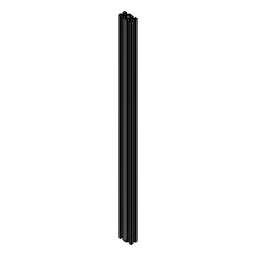
drawing-machine (Autodesk Fusion 360 archive; units mm, degrees)
design "40x20 extrusion"
Autodesk Fusion 360 part; units mm, degrees
sketch "Sketch1" plane through (0, 0, 0) normal (0, 0, 1) x (1, 0, 0)
  line L0 (20, -10) -> (-20, -10) construction
  line L1 (-20, -10) -> (-20, 10) construction
  line L2 (-20, 10) -> (20, 10) construction
  line L3 (20, 10) -> (20, -10) construction
  line L4 (20, -10) -> (-20, 10) construction
  line L5 (-20, -10) -> (20, 10) construction
  line L6 (0, -10) -> (0, 10) construction
  line L7 (-20, 0) -> (0, 0) construction
  circle A0 centre (-10, 0) radius 2.5
  line L8 (-6.1, -3.9) -> (-13.9, -3.9)
  line L9 (-13.9, -3.9) -> (-13.9, 3.9)
  line L10 (-13.9, 3.9) -> (-6.1, 3.9)
  line L11 (-6.1, 3.9) -> (-6.1, -3.9)
  line L12 (-6.1, -3.9) -> (-13.9, 3.9) construction
  line L13 (-13.9, -3.9) -> (-6.1, 3.9) construction
  circle A1 centre (-19.1, 9.1) radius 0.9
  line L14 (-19.1, 10) -> (-13.45, 10)
  line L15 (0, 10) -> (-5.65, 10) construction
  line L16 (-5.65, 10) -> (-13.45, 10) construction
  line L17 (-13.45, 10) -> (-13.45, 8.07) construction
  line L18 (-9.55, 10) -> (-9.55, 8.07) construction
  line L19 (-15.05, 8.07) -> (-4.05, 8.07) construction
  line L20 (-13.9, 3.9) -> (-19.1, 9.1) construction
  line L21 (-9.55, 10) -> (-9.55, 8.87) construction
  line L22 (-6.45, 8.87) -> (-12.65, 8.87) construction
  line L23 (-12.65, 8.87) -> (-13.45, 10)
  line L24 (-12.65, 8.87) -> (-12.65, 8.07)
  line L25 (-15.05, 8.07) -> (-12.65, 8.07)
  line L26 (-11.7787, 3.9) -> (-15.05, 7.1713)
  line L27 (-15.05, 7.1713) -> (-15.05, 8.07)
  line L28 (-13.9, 1.7787) -> (-17.1713, 5.05)
  line L29 (-18.07, 5.05) -> (-18.07, 2.65)
  line L30 (-18.87, 2.65) -> (-18.07, 2.65)
  line L31 (-18.87, 2.65) -> (-20, 3.45)
  line L32 (-20, 9.1) -> (-20, 3.45)
  line L33 (-17.1713, 5.05) -> (-18.07, 5.05)
  line L34 (15.05, 8.07) -> (12.65, 8.07)
  line L35 (15.05, 7.1713) -> (15.05, 8.07)
  line L36 (11.7787, 3.9) -> (15.05, 7.1713)
  line L37 (13.9, 1.7787) -> (17.1713, 5.05)
  line L38 (17.1713, 5.05) -> (18.07, 5.05)
  line L39 (18.07, 5.05) -> (18.07, 2.65)
  line L40 (18.87, 2.65) -> (18.07, 2.65)
  line L41 (18.87, 2.65) -> (20, 3.45)
  line L42 (20, 9.1) -> (20, 3.45)
  circle A2 centre (19.1, 9.1) radius 0.9
  line L43 (19.1, 10) -> (13.45, 10)
  line L44 (12.65, 8.87) -> (13.45, 10)
  line L45 (12.65, 8.87) -> (12.65, 8.07)
  line L46 (13.9, -1.7787) -> (17.1713, -5.05)
  line L47 (17.1713, -5.05) -> (18.07, -5.05)
  line L48 (18.07, -5.05) -> (18.07, -2.65)
  line L49 (18.87, -2.65) -> (18.07, -2.65)
  line L50 (18.87, -2.65) -> (20, -3.45)
  line L51 (20, -9.1) -> (20, -3.45)
  circle A3 centre (19.1, -9.1) radius 0.9
  line L52 (19.1, -10) -> (13.45, -10)
  line L53 (12.65, -8.87) -> (13.45, -10)
  line L54 (12.65, -8.87) -> (12.65, -8.07)
  line L55 (15.05, -8.07) -> (12.65, -8.07)
  line L56 (11.7787, -3.9) -> (15.05, -7.1713)
  line L57 (15.05, -7.1713) -> (15.05, -8.07)
  line L58 (-13.9, -1.7787) -> (-17.1713, -5.05)
  line L59 (-17.1713, -5.05) -> (-18.07, -5.05)
  line L60 (-18.07, -5.05) -> (-18.07, -2.65)
  line L61 (-18.87, -2.65) -> (-18.07, -2.65)
  line L62 (-18.87, -2.65) -> (-20, -3.45)
  line L63 (-20, -9.1) -> (-20, -3.45)
  circle A4 centre (-19.1, -9.1) radius 0.9
  line L64 (-19.1, -10) -> (-13.45, -10)
  line L65 (-12.65, -8.87) -> (-13.45, -10)
  line L66 (-12.65, -8.87) -> (-12.65, -8.07)
  line L67 (-15.05, -8.07) -> (-12.65, -8.07)
  line L68 (-11.7787, -3.9) -> (-15.05, -7.1713)
  line L69 (-15.05, -7.1713) -> (-15.05, -8.07)
  line L70 (6.1, 3.9) -> (6.1, -3.9)
  line L71 (6.1, -3.9) -> (13.9, -3.9)
  line L72 (13.9, -3.9) -> (13.9, 3.9)
  line L73 (13.9, 3.9) -> (6.1, 3.9)
  circle A5 centre (10, 0) radius 2.5
  line L74 (10, 3.9) -> (10, -3.9) construction
  line L75 (6.1, 3.9) -> (0, 10) construction
  line L76 (6.1, 1.7787) -> (0.7076, 7.1711)
  line L77 (8.2213, 3.9) -> (4.9502, 7.1711)
  line L78 (0.7076, 7.1711) -> (0.7076, 8.0701)
  line L79 (0.7076, 7.1711) -> (4.9502, 7.1711) construction
  line L80 (4.9502, 7.1711) -> (4.9502, 8.0701)
  line L81 (0.7076, 8.0701) -> (0, 8.0701)
  line L82 (4.9502, 8.0701) -> (7.3502, 8.0701)
  line L83 (7.3502, 8.0701) -> (7.3502, 10)
  line L84 (7.3502, 10) -> (0, 10)
  line L85 (6.55, 10) -> (7.3502, 8.8701)
  line L86 (-6.1, 1.7787) -> (-0.7076, 7.1711)
  line L87 (-0.7076, 7.1711) -> (-0.7076, 8.0701)
  line L88 (-0.7076, 8.0701) -> (0, 8.0701)
  line L89 (-8.2213, 3.9) -> (-4.9502, 7.1711)
  line L90 (-4.9502, 7.1711) -> (-4.9502, 8.0701)
  line L91 (-4.9502, 8.0701) -> (-7.3502, 8.0701)
  line L92 (-6.55, 10) -> (-7.3502, 8.8701)
  line L93 (-7.3502, 8.0701) -> (-7.3502, 10)
  line L94 (-7.3502, 10) -> (0, 10)
  line L95 (-6.1, -1.7787) -> (-0.7076, -7.1711)
  line L96 (-0.7076, -7.1711) -> (-0.7076, -8.0701)
  line L97 (-0.7076, -8.0701) -> (0, -8.0701)
  line L98 (0.7076, -8.0701) -> (0, -8.0701)
  line L99 (6.1, -1.7787) -> (0.7076, -7.1711)
  line L100 (0.7076, -7.1711) -> (0.7076, -8.0701)
  line L101 (8.2213, -3.9) -> (4.9502, -7.1711)
  line L102 (4.9502, -7.1711) -> (4.9502, -8.0701)
  line L103 (4.9502, -8.0701) -> (7.3502, -8.0701)
  line L104 (6.55, -10) -> (7.3502, -8.8701)
  line L105 (7.3502, -8.0701) -> (7.3502, -10)
  line L106 (7.3502, -10) -> (0, -10)
  line L107 (-4.9502, -7.1711) -> (-4.9502, -8.0701)
  line L108 (-8.2213, -3.9) -> (-4.9502, -7.1711)
  line L109 (-4.9502, -8.0701) -> (-7.3502, -8.0701)
  line L110 (-6.55, -10) -> (-7.3502, -8.8701)
  line L111 (-7.3502, -8.0701) -> (-7.3502, -10)
  line L112 (-7.3502, -10) -> (0, -10)
  point P0 (-10, 0)
  dimension "d1" = 40
  dimension "d2" = 20
  dimension "d3" = 5
  dimension "d4" = 7.8
  dimension "d5" = 7.8
  dimension "d6" = 1.8
  dimension "d7" = 1.93
  dimension "d8" = 11
  dimension "d9" = 6.2
  dimension "d10" = 0.8
  dimension "d12" = 1.5
  dimension "d13" = 1.5
  dimension "d14" = 1.5
  dimension "d15" = 4.626
  dimension "d16" = 0.899
  dimension "d17" = 2.4
  dimension "d18" = 0.8
  dimension "d19" = 6.55
  constraint horizontal L0
  constraint perpendicular L0 L1
  constraint parallel L0 L2
  constraint parallel L1 L3
  constraint coincident L4 L7.end
  constraint coincident L5 L7.end
  constraint coincident L7.end origin
  constraint midpoint L0 L6.start
  constraint midpoint L2 L6.end
  constraint midpoint L1 L7.start
  constraint midpoint L7 P0
  constraint horizontal L8
  constraint perpendicular L8 L9
  constraint parallel L8 L10
  constraint parallel L9 L11
  constraint coincident L12 P0
  constraint coincident L13 P0
  constraint coincident P0 A0.centre
  constraint tangent L2 A1
  constraint tangent L1 A1
  constraint coincident A1 L14.start
  constraint coincident L2 L14.start
  constraint coincident L2 L14.end
  constraint tangent A1 L14
  constraint coincident L2 L15.end
  constraint equal L14 L15
  constraint equal L10 L16
  constraint perpendicular L16 L17
  constraint midpoint L16 L18.start
  constraint perpendicular L2 L18
  constraint perpendicular L18 L19
  constraint midpoint L18.end L19
  constraint coincident L17.end L19
  constraint parallel L12 L20
  constraint coincident L18 L21.end
  constraint perpendicular L2 L21
  constraint parallel L19 L22
  constraint midpoint L21.end L22
  constraint coincident L19 L24.end
  constraint perpendicular L19 L24
  constraint coincident L10 L26.start
  constraint perpendicular L19 L27
  constraint parallel L20 L26
  constraint symmetric L14.start L20 L32.start
  constraint symmetric L14.end L20 L31.end
  constraint symmetric L19.start L20 L29.start
  constraint symmetric L20 L22.end L30.start
  constraint symmetric L20 L24.end L29.end
  constraint symmetric L20 L26.start L28.start
  constraint symmetric L20 L26.end L28.end
  constraint symmetric L6 A1 A2
  constraint symmetric L6 L14.start L43.start
  constraint symmetric L6 L14.end L43.end
  constraint symmetric L6 L19.start L34.start
  constraint symmetric L6 L22.end L44.start
  constraint symmetric L6 L24.end L34.end
  constraint symmetric L6 L26.start L36.start
  constraint symmetric L6 L26.end L35.start
  constraint symmetric L6 L28.start L37.start
  constraint symmetric L6 L28.end L37.end
  constraint symmetric L6 L29.start L38.end
  constraint symmetric L6 L29.end L39.end
  constraint symmetric L6 L30.start L40.start
  constraint symmetric L6 L31.end L41.end
  constraint symmetric L6 L32.start L42.start
  constraint symmetric L7 A1 A4
  constraint symmetric L7 L14.start L64.start
  constraint symmetric L7 L14.end L64.end
  constraint symmetric L7 L19.start L67.start
  constraint symmetric L7 L22.end L65.start
  constraint symmetric L7 L24.end L66.end
  constraint symmetric L7 L26.start L68.start
  constraint symmetric L7 L26.end L68.end
  constraint symmetric L7 L28.start L58.start
  constraint symmetric L7 L28.end L58.end
  constraint symmetric L7 L29.start L59.end
  constraint symmetric L7 L29.end L60.end
  constraint symmetric L7 L30.start L61.start
  constraint symmetric L7 L31.end L62.end
  constraint symmetric L7 L32.start L63.start
  constraint symmetric L7 L34.start L55.start
  constraint symmetric L7 L34.end L54.end
  constraint symmetric L7 L35.start L56.end
  constraint symmetric L7 L36.start L56.start
  constraint symmetric L7 L37.start L46.start
  constraint symmetric L7 L37.end L46.end
  constraint symmetric L7 L38.end L47.end
  constraint symmetric L7 L39.end L48.end
  constraint symmetric L7 L40.start L49.start
  constraint symmetric L7 L41.end L50.end
  constraint symmetric L7 L42.start L51.start
  constraint symmetric L7 A2 A3
  constraint symmetric L7 L43.start L52.start
  constraint symmetric L7 L43.end L52.end
  constraint symmetric L7 L44.start L53.start
  constraint symmetric L6 A0 A5
  constraint symmetric L6 L8.start L70.end
  constraint symmetric L6 L8.end L71.end
  constraint symmetric L6 L9.end L72.end
  constraint symmetric L6 L10.end L70.start
  constraint midpoint L73 L74.start
  constraint midpoint L71 L74.end
  constraint coincident L6 L15.start
  constraint parallel L20 L75
  constraint coincident L70 L76.start
  constraint parallel L75 L76
  constraint coincident L73 L77.start
  constraint parallel L75 L77
  constraint vertical L78
  constraint parallel L73 L79
  constraint perpendicular L79 L80
  constraint equal L78 L80
  constraint coincident L6 L81.end
  constraint perpendicular L6 L81
  constraint perpendicular L80 L82
  constraint coincident L2 L83.end
  constraint perpendicular L2 L83
  constraint coincident L2 L85.start
  constraint coincident L83 L85.end
  constraint symmetric L15.start L6 L75.end
  constraint symmetric L6 L76.start L86.start
  constraint symmetric L6 L76.end L86.end
  constraint symmetric L6 L77.start L89.start
  constraint symmetric L6 L77.end L89.end
  constraint symmetric L6 L78.end L87.end
  constraint symmetric L6 L80.end L90.end
  constraint symmetric L6 L81.end L88.end
  constraint symmetric L6 L82.end L91.end
  constraint symmetric L6 L83.end L93.end
  constraint symmetric L6 L85.start L92.start
  constraint symmetric L6 L85.end L92.end
  constraint symmetric L6.end L7 L6.start
  constraint symmetric L7 L76.start L99.start
  constraint symmetric L7 L76.end L99.end
  constraint symmetric L7 L77.start L101.start
  constraint symmetric L7 L77.end L101.end
  constraint symmetric L7 L78.end L98.start
  constraint symmetric L7 L80.end L102.end
  constraint symmetric L7 L81.end L97.end
  constraint symmetric L7 L82.end L103.end
  constraint symmetric L7 L83.end L105.end
  constraint symmetric L7 L85.start L104.start
  constraint symmetric L7 L85.end L104.end
  constraint symmetric L7 L86.start L95.start
  constraint symmetric L7 L86.end L95.end
  constraint symmetric L7 L87.end L96.end
  constraint symmetric L7 L89.start L108.start
  constraint symmetric L7 L89.end L107.start
  constraint symmetric L7 L90.end L107.end
  constraint symmetric L7 L91.end L109.end
  constraint symmetric L7 L92.start L110.start
  constraint symmetric L7 L92.end L110.end
  constraint symmetric L7 L93.end L111.end
  constraint symmetric L7 L6.end L6.start
  measures "d1" distance of L1.end L2.end
  measures "d2" distance of L0.end L1.end
  measures "d3" diameter of A0
  measures "d4" distance of L9.end L10.end L22
  measures "d5" distance of L8.end L9.end
  measures "d6" diameter of A1
  measures "d7" distance of L14.end L17.end
  measures "d8" distance of L19.start L19.end
  measures "d9" distance of L22.start L22.end
  measures "d10" distance of L19 L22
  measures "d12" distance of L20 L26
  measures "d13" distance of L75 L77
  measures "d14" distance of L75 L76
  measures "d15" distance of L77.start L77.end
  measures "d16" distance of L76.end L78.end
  measures "d17" distance of L80.end L82.end
  measures "d18" distance of L82.end L85.end
  measures "d19" distance of L6.end L85.start
extrude "Extrude1" add sketch "Sketch1" along normal blind 600 contours L8 L11 L70 L71 L95 L96 L97 L98 L99 L100 L101 L102 L103 L104 L105 L106 L107 L108 L109 L110 L111 L112 | L8 L9 L10 L11 | L8 L9 L58 L59 L60 L61 L62 L63 A4 L64 L65 L66 L67 L68 L69 | L10 L11 L70 L73 L76 L77 L78 L80 L81 L82 L83 L84 L85 L86 L87 L88 L89 L90 L91 L92 L93 L94 | L9 L10 A1 L14 L23 L24 L25 L26 L27 L28 L29 L30 L31 L32 L33 | L70 L71 L72 L73 | A4 | L46 L47 L48 L49 L50 L51 A3 L52 L53 L54 L55 L56 L57 L71 L72 | A1 | L34 L35 L36 L37 L38 L39 L40 L41 L42 A2 L43 L44 L45 L72 L73 | A3 | A2
sketch "Sketch2" plane through (0, 0, 0) normal (0, 0, -1) x (1, 0, 0)
  circle A0 centre (10, 0) radius 2.5
  circle A1 centre (-10, 0) radius 2.5
  line L0 (6.1, -1.7787) -> (0.7076, -7.1711)
  line L1 (0.7076, -7.1711) -> (0.7076, -8.0701)
  line L2 (0.7076, -8.0701) -> (-0.7076, -8.0701)
  line L3 (-0.7076, -8.0701) -> (-0.7076, -7.1711)
  line L4 (-0.7076, -7.1711) -> (-6.1, -1.7787)
  line L5 (-6.1, -1.7787) -> (-6.1, 1.7787)
  line L6 (-6.1, 1.7787) -> (-0.7076, 7.1711)
  line L7 (-0.7076, 7.1711) -> (-0.7076, 8.0701)
  line L8 (-0.7076, 8.0701) -> (0.7076, 8.0701)
  line L9 (0.7076, 8.0701) -> (0.7076, 7.1711)
  line L10 (0.7076, 7.1711) -> (6.1, 1.7787)
  line L11 (6.1, 1.7787) -> (6.1, -1.7787)
  line L12 (7.3502, 8.8701) -> (6.55, 10)
  line L13 (6.55, 10) -> (-6.55, 10)
  line L14 (-6.55, 10) -> (-7.3502, 8.8701)
  line L15 (-7.3502, 8.8701) -> (-7.3502, 8.0701)
  line L16 (-7.3502, 8.0701) -> (-4.9502, 8.0701)
  line L17 (-4.9502, 8.0701) -> (-4.9502, 7.1711)
  line L18 (-4.9502, 7.1711) -> (-8.2213, 3.9)
  line L19 (-8.2213, 3.9) -> (-11.7787, 3.9)
  line L20 (-11.7787, 3.9) -> (-15.05, 7.1713)
  line L21 (-15.05, 7.1713) -> (-15.05, 8.07)
  line L22 (-15.05, 8.07) -> (-12.65, 8.07)
  line L23 (-12.65, 8.07) -> (-12.65, 8.87)
  line L24 (-12.65, 8.87) -> (-13.45, 10)
  line L25 (-13.45, 10) -> (-19.1, 10)
  arc A2 (-19.1, 10) -> (-20, 9.1) centre (-19.1, 9.1) ccw
  line L26 (-20, 9.1) -> (-20, 3.45)
  line L27 (-20, 3.45) -> (-18.87, 2.65)
  line L28 (-18.87, 2.65) -> (-18.07, 2.65)
  line L29 (-18.07, 2.65) -> (-18.07, 5.05)
  line L30 (-18.07, 5.05) -> (-17.1713, 5.05)
  line L31 (-17.1713, 5.05) -> (-13.9, 1.7787)
  line L32 (-13.9, 1.7787) -> (-13.9, -1.7787)
  line L33 (-13.9, -1.7787) -> (-17.1713, -5.05)
  line L34 (-17.1713, -5.05) -> (-18.07, -5.05)
  line L35 (-18.07, -5.05) -> (-18.07, -2.65)
  line L36 (-18.07, -2.65) -> (-18.87, -2.65)
  line L37 (-18.87, -2.65) -> (-20, -3.45)
  line L38 (-20, -3.45) -> (-20, -9.1)
  arc A3 (-20, -9.1) -> (-19.1, -10) centre (-19.1, -9.1) ccw
  line L39 (-19.1, -10) -> (-13.45, -10)
  line L40 (-13.45, -10) -> (-12.65, -8.87)
  line L41 (-12.65, -8.87) -> (-12.65, -8.07)
  line L42 (-12.65, -8.07) -> (-15.05, -8.07)
  line L43 (-15.05, -8.07) -> (-15.05, -7.1713)
  line L44 (-15.05, -7.1713) -> (-11.7787, -3.9)
  line L45 (-11.7787, -3.9) -> (-8.2213, -3.9)
  line L46 (-8.2213, -3.9) -> (-4.9502, -7.1711)
  line L47 (-4.9502, -7.1711) -> (-4.9502, -8.0701)
  line L48 (-4.9502, -8.0701) -> (-7.3502, -8.0701)
  line L49 (-7.3502, -8.0701) -> (-7.3502, -8.8701)
  line L50 (-7.3502, -8.8701) -> (-6.55, -10)
  line L51 (-6.55, -10) -> (6.55, -10)
  line L52 (6.55, -10) -> (7.3502, -8.8701)
  line L53 (7.3502, -8.8701) -> (7.3502, -8.0701)
  line L54 (7.3502, -8.0701) -> (4.9502, -8.0701)
  line L55 (4.9502, -8.0701) -> (4.9502, -7.1711)
  line L56 (4.9502, -7.1711) -> (8.2213, -3.9)
  line L57 (8.2213, -3.9) -> (11.7787, -3.9)
  line L58 (11.7787, -3.9) -> (15.05, -7.1713)
  line L59 (15.05, -7.1713) -> (15.05, -8.07)
  line L60 (15.05, -8.07) -> (12.65, -8.07)
  line L61 (12.65, -8.07) -> (12.65, -8.87)
  line L62 (12.65, -8.87) -> (13.45, -10)
  line L63 (13.45, -10) -> (19.1, -10)
  arc A4 (19.1, -10) -> (20, -9.1) centre (19.1, -9.1) ccw
  line L64 (20, -9.1) -> (20, -3.45)
  line L65 (20, -3.45) -> (18.87, -2.65)
  line L66 (18.87, -2.65) -> (18.07, -2.65)
  line L67 (18.07, -2.65) -> (18.07, -5.05)
  line L68 (18.07, -5.05) -> (17.1713, -5.05)
  line L69 (17.1713, -5.05) -> (13.9, -1.7787)
  line L70 (13.9, -1.7787) -> (13.9, 1.7787)
  line L71 (13.9, 1.7787) -> (17.1713, 5.05)
  line L72 (17.1713, 5.05) -> (18.07, 5.05)
  line L73 (18.07, 5.05) -> (18.07, 2.65)
  line L74 (18.07, 2.65) -> (18.87, 2.65)
  line L75 (18.87, 2.65) -> (20, 3.45)
  line L76 (20, 3.45) -> (20, 9.1)
  arc A5 (20, 9.1) -> (19.1, 10) centre (19.1, 9.1) ccw
  line L77 (19.1, 10) -> (13.45, 10)
  line L78 (13.45, 10) -> (12.65, 8.87)
  line L79 (12.65, 8.87) -> (12.65, 8.07)
  line L80 (12.65, 8.07) -> (15.05, 8.07)
  line L81 (15.05, 8.07) -> (15.05, 7.1713)
  line L82 (15.05, 7.1713) -> (11.7787, 3.9)
  line L83 (11.7787, 3.9) -> (8.2213, 3.9)
  line L84 (8.2213, 3.9) -> (4.9502, 7.1711)
  line L85 (4.9502, 7.1711) -> (4.9502, 8.0701)
  line L86 (4.9502, 8.0701) -> (7.3502, 8.0701)
  line L87 (7.3502, 8.0701) -> (7.3502, 8.8701)
  line L88 (0, 10) -> (0, -10)
  constraint midpoint L13 L88.start
  constraint midpoint L51 L88.end
equation "d20 = Length"
equation "Length = 600 mm"

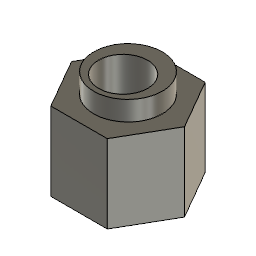
design "eccentric nut"
Autodesk Fusion 360 part; units mm, degrees
sketch "Sketch1" plane through (0, 0, 0) normal (0, 0, 1) x (1, 0, 0)
  line L0 (2.8868, -5) -> (5.7735, 0)
  line L1 (5.7735, 0) -> (2.8868, 5)
  line L2 (2.8868, 5) -> (-2.8868, 5)
  line L3 (-2.8868, 5) -> (-5.7735, 0)
  line L4 (-5.7735, 0) -> (-2.8868, -5)
  line L5 (-2.8868, -5) -> (2.8868, -5)
  dimension "d1" = 10
  constraint horizontal L2
  measures "d1" distance of L2 L5
extrude "Extrude1" add sketch "Sketch1" along normal blind 8
sketch "Sketch2" plane through (0, 0, 8) normal (0, 0, 1) x (-1, 0, 0)
  line L0 (2.8868, 5) -> (-2.8868, 5)
  line L1 (-2.8868, 5) -> (-5.7735, 0)
  line L2 (-5.7735, 0) -> (-2.8868, -5)
  line L3 (-2.8868, -5) -> (2.8868, -5)
  line L4 (2.8868, -5) -> (5.7735, 0)
  line L5 (5.7735, 0) -> (2.8868, 5)
  circle A0 centre (0, 0) radius 3.5
  dimension "d4" = 7
  constraint coincident A0.centre origin
  measures "d4" diameter of A0
extrude "Extrude2" add sketch "Sketch2" along normal blind 2 contours A0
sketch "Sketch4" plane through (0, 0, 10) normal (0, 0, 1) x (-1, 0, 0)
  circle A0 centre (0, 0) radius 3.5
  line L0 (0, 0) -> (0, 0.5) construction
  circle A1 centre (0, 0.5) radius 2.5
  dimension "d8" = 0.5
  dimension "d9" = 5
  constraint coincident A0.centre L0.start
  constraint vertical L0
  constraint coincident L0.end A1.centre
  measures "d8" distance of A0.centre L0.end
  measures "d9" diameter of A1
extrude "Extrude3" cut sketch "Sketch4" against normal up to surface (10 mm away) contours A1

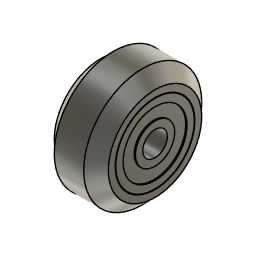
design "PP_TRNS_V-Wheel"
Autodesk Fusion 360 part; units mm, degrees
sketch "Sketch1" plane through (0, 0, 0) normal (0, 1, 0) x (1, 0, 0)
  line L0 (0, -12) -> (0, -2.5)
  line L1 (0, -12) -> (3, -12)
  line L2 (3, -12) -> (5.5, -9.5)
  line L3 (5.5, -9.5) -> (5.5, -8.1)
  line L4 (5.5, -8.1) -> (5.25, -8.1)
  line L5 (5.25, -8.1) -> (5.25, -8)
  line L6 (5.25, -8) -> (5.5, -8)
  line L7 (5.5, -8) -> (5.5, -6.5)
  line L8 (5.5, -6.5) -> (5.25, -6.5)
  line L9 (5.25, -6.5) -> (5.25, -4)
  line L10 (5.25, -4) -> (5.5, -4)
  line L11 (5.5, -4) -> (5.5, -2.5)
  line L12 (5.5, -2.5) -> (0, -2.5)
  dimension "d1" = 2.5
  dimension "d2" = 12
  dimension "d3" = 5.5
  dimension "d4" = 1.5
  dimension "d5" = 1.5
  dimension "d6" = 0.25
  dimension "d7" = 3
  dimension "d8" = 0.1
  dimension "d9" = 8
  dimension "d10" = 45
  constraint vertical L0
  constraint perpendicular L0 L1
  constraint perpendicular L1 L3
  constraint perpendicular L3 L4
  constraint perpendicular L4 L5
  constraint perpendicular L5 L6
  constraint perpendicular L4 L7
  constraint perpendicular L7 L8
  constraint perpendicular L8 L9
  constraint perpendicular L9 L10
  constraint perpendicular L8 L11
  constraint perpendicular L11 L12
  constraint coincident origin L0
  constraint coincident L7 L10.end
  constraint coincident L5 L8.end
  constraint coincident L3 L6.end
  measures "d1" distance of origin L12
  measures "d2" distance of origin L0.start
  measures "d3" distance of L11.end L0.end
  measures "d4" distance of L10.end L11.end
  measures "d5" distance of L6.end L7.end
  measures "d6" distance of L9.end L10.end
  measures "d7" distance of L0.start L1.end
  measures "d8" distance of L4.end L5.end
  measures "d9" vertical distance of origin L6.end
  measures "d10" angle of L1 L2
revolve "Revolve1" add sketch "Sketch1" angle 360 about axis through (1.75, 0, 0) along (1, 0, 0)
mirror "Mirror1" about plane through (0, 0, 0) normal (1, 0, 0) of bodies 1 merged
equation "d2 = ( 24 / 2 ) * 1 mm"
equation "d3 = ( 11 / 2 ) * 1 mm"
equation "d7 = ( 6 / 2 ) * 1 mm"

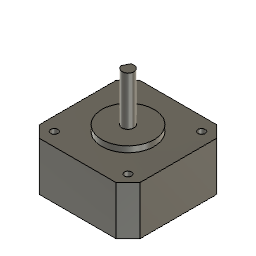
design "Nema 17 Short"
Autodesk Fusion 360 part; units mm, degrees
sketch "Sketch1" plane through (0, 0, 0) normal (0, 0, 1) x (1, 0, 0)
  line L0 (21.15, -21.15) -> (-21.15, -21.15)
  line L1 (-21.15, -21.15) -> (-21.15, 21.15)
  line L2 (-21.15, 21.15) -> (21.15, 21.15)
  line L3 (21.15, 21.15) -> (21.15, -21.15)
  line L4 (21.15, -21.15) -> (-21.15, 21.15) construction
  line L5 (-21.15, -21.15) -> (21.15, 21.15) construction
  dimension "d1" = 42.3
  constraint horizontal L0
  constraint perpendicular L0 L1
  constraint parallel L0 L2
  constraint parallel L1 L3
  constraint coincident L4 origin
  constraint coincident L5 origin
  constraint equal L2 L3
  measures "d1" distance of L1.end L2.end
extrude "Extrude1" add sketch "Sketch1" along normal blind 20.5 makes body 1
sketch "Sketch2" plane through (0, 0, 20.5) normal (0, 0, 1) x (-1, 0, 0)
  line L0 (-21.15, -21.15) -> (21.15, -21.15)
  line L1 (21.15, -21.15) -> (21.15, 21.15)
  line L2 (21.15, 21.15) -> (-21.15, 21.15)
  line L3 (-21.15, 21.15) -> (-21.15, -21.15)
  circle A0 centre (0, 0) radius 11
  dimension "d4" = 22
  constraint coincident A0.centre origin
  measures "d4" diameter of A0
extrude "Extrude2" add sketch "Sketch2" along normal blind 2.5 contours A0 bodies 1
sketch "Sketch3" plane through (0, 0, 23) normal (0, 0, 1) x (-1, 0, 0)
  circle A0 centre (0, 0) radius 11
  circle A1 centre (0, 0) radius 2.5
  line L0 (1.5, 2) -> (-1.5, 2)
  line L1 (0, 2) -> (0, -2.5) construction
  dimension "d7" = 4.5
  dimension "d8" = 5
  constraint coincident A0.centre A1.centre
  constraint coincident A1 L0.start
  constraint coincident A1 L0.end
  constraint horizontal L0
  constraint midpoint L0 L1.start
  constraint coincident A1 L1.end
  constraint perpendicular L0 L1
  measures "d7" distance of L1.start L1.end
  measures "d8" diameter of A1
extrude "Extrude3" add sketch "Sketch3" along normal blind 20.5 contours A1 L0 picked at (0.8123, -0.6533) bodies 1
extrude "Extrude4" add sketch "Sketch3" along normal blind 1.5 contours A1 L0 picked at (0.0487, 2.343) bodies 1
chamfer "Chamfer1" distance 5 angle 45 4 edges at (21.15, -21.15, 10.25) (21.15, 21.15, 10.25) (-21.15, 21.15, 10.25) (-21.15, -21.15, 10.25) on bodies 1
sketch "Sketch4" plane through (0, 0, 20.5) normal (0, 0, 1) x (-1, 0, 0)
  line L0 (21.15, 16.15) -> (16.15, 21.15)
  line L1 (16.15, 21.15) -> (-16.15, 21.15)
  line L2 (-16.15, 21.15) -> (-21.15, 16.15)
  line L3 (-21.15, 16.15) -> (-21.15, -16.15)
  line L4 (-21.15, -16.15) -> (-16.15, -21.15)
  line L5 (-16.15, -21.15) -> (16.15, -21.15)
  line L6 (16.15, -21.15) -> (21.15, -16.15)
  line L7 (21.15, -16.15) -> (21.15, 16.15)
  circle A0 centre (0, 0) radius 11
  line L8 (-15.5, 15.5) -> (15.5, 15.5) construction
  line L9 (15.5, 15.5) -> (15.5, -15.5) construction
  line L10 (15.5, -15.5) -> (-15.5, -15.5) construction
  line L11 (-15.5, -15.5) -> (-15.5, 15.5) construction
  line L12 (-15.5, 15.5) -> (15.5, -15.5) construction
  line L13 (15.5, 15.5) -> (-15.5, -15.5) construction
  circle A1 centre (15.5, -15.5) radius 1.5
  circle A2 centre (-15.5, -15.5) radius 1.5
  circle A3 centre (-15.5, 15.5) radius 1.5
  circle A4 centre (15.5, 15.5) radius 1.5
  dimension "d14" = 3
  dimension "d15" = 31
  constraint horizontal L8
  constraint perpendicular L8 L9
  constraint parallel L8 L10
  constraint parallel L9 L11
  constraint coincident L12 A0.centre
  constraint coincident L13 A0.centre
  constraint coincident A0.centre origin
  constraint coincident L9.end L10.start
  constraint coincident L10.end L11.start
  constraint coincident L8.start L11.end
  constraint coincident L8.end L9.start
  constraint equal A2 A3
  constraint equal A3 A4
  constraint equal A1 A4
  constraint equal L9 L10
  measures "d14" diameter of A1
  measures "d15" distance of L9.end L10.end
extrude "Extrude5" cut sketch "Sketch4" against normal blind 5 contours A1 | A2 | A3 | A4 bodies 1
split "Split1" by plane through (0, 0, 23) normal (0, 0, 1) bodies 1 makes body 2 at (-1.6901, -1.8422, 30.3333)
copy_body "Body->Comp1" bodies 2 removing the originals makes body 3 in component "shaft"
copy_body "Body->Comp2" bodies 1 removing the originals makes body 4 in component "body"
component "shaft" placed x (1, 0, 0) y (0, 1, 0) z (0, 0, 1) at (0, 0, 0)
component "body" placed x (1, 0, 0) y (0, 1, 0) z (0, 0, 1) at (0, 0, 0)
named bodies: "body", "shaft"

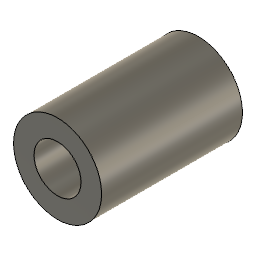
design "linear bearing"
Autodesk Fusion 360 part; units mm, degrees
sketch "Sketch1" plane through (0, 0, 0) normal (0, 1, 0) x (1, 0, 0)
  circle A0 centre (0, 0) radius 4
  circle A1 centre (0, 0) radius 7.5
  dimension "d1" = 8
  dimension "d2" = 15
  constraint coincident A0.centre A1.centre
  measures "d1" diameter of A0
  measures "d2" diameter of A1
extrude "Extrude1" add sketch "Sketch1" along normal blind 24

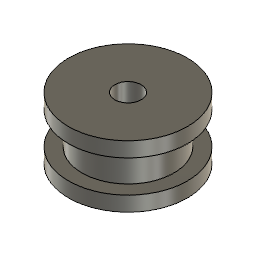
design "belt idler"
Autodesk Fusion 360 part; units mm, degrees
sketch "Sketch1" plane through (0, 0, 0) normal (0, 0, 1) x (1, 0, 0)
  circle A0 centre (0, 0) radius 12
  dimension "d1" = 24
  constraint coincident A0.centre origin
  measures "d1" diameter of A0
extrude "Extrude1" add sketch "Sketch1" along normal blind 3
sketch "Sketch5" plane through (0, 0, 0) normal (0, 0, -1) x (1, 0, 0)
  circle A0 centre (0, 0) radius 12
  circle A1 centre (0, 0) radius 4
  circle A2 centre (0, 0) radius 9.25
  dimension "d13" = 8
  dimension "d14" = 18.5
  constraint coincident A0.centre A1.centre
  measures "d13" diameter of A1
  measures "d14" diameter of A2
extrude "Extrude5" add sketch "Sketch5" along normal blind 6.5 contours A2
sketch "Sketch6" plane through (0, 0, -6.5) normal (0, 0, -1) x (1, 0, 0)
  circle A0 centre (0, 0) radius 4
  circle A1 centre (0, 0) radius 9.25
  circle A2 centre (0, 0) radius 12
  circle A3 centre (0, 0) radius 9.25
extrude "Extrude6" add sketch "Sketch6" along normal blind 3 contours A1 A3 | A2
sketch "Sketch7" plane through (0, 0, 0) normal (0, 0, -1) x (1, 0, 0)
  circle A0 centre (0, 0) radius 4
  circle A1 centre (0, 0) radius 2.65
  dimension "d19" = 5.3
  constraint coincident A0.centre A1.centre
  measures "d19" diameter of A1
extrude "Extrude7" cut sketch "Sketch7" against normal up to surface (3 mm away) contours A1
ref_plane "WorkPlane1" through (0, 0, -3.25) normal (0, 0, -1) x (1, 0, 0)
extrude "Extrude8" add 1 faces at (3.5351, 0.1987, 0) along direction (0, 0, -1) up to surface (2 mm away)

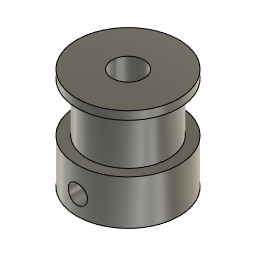
design "PP_TRNS_GT2-Pulley-20T-6mm"
Autodesk Fusion 360 part; units mm, degrees
sketch "Sketch1" plane through (0, 0, 0) normal (0, 1, 0) x (1, 0, 0)
  line L0 (0, 0) -> (8, 0)
  line L1 (8, 0) -> (8, -7)
  line L2 (8, -7) -> (6.3662, -7)
  line L3 (6.3662, -7) -> (6.3662, -14.7)
  line L4 (6.3662, -14.7) -> (8, -14.7)
  line L5 (8, -14.7) -> (8, -16)
  line L6 (8, -16) -> (2.5, -16)
  line L7 (2.5, -16) -> (2.5, 0)
  circle A0 centre (0, -3) radius 1.5
  line L8 (0, 0) -> (0, -3) construction
  dimension "d1" = 2.5
  dimension "d2" = 8
  dimension "d3" = 7
  dimension "d4" = 6.3662
  dimension "d5" = 1.3
  dimension "d6" = 16
  dimension "d8" = 3
  dimension "d9" = 3
  constraint coincident L0.start L8.start
  constraint horizontal L0
  constraint perpendicular L0 L1
  constraint perpendicular L1 L2
  constraint perpendicular L2 L3
  constraint perpendicular L3 L4
  constraint perpendicular L4 L5
  constraint perpendicular L3 L6
  constraint coincident L0 L7.end
  constraint perpendicular L0 L7
  constraint coincident L1.end L5
  constraint coincident A0.centre L8.end
  constraint vertical L8
  measures "d1" distance of L0.start L7
  measures "d2" distance of L0.start L1
  measures "d3" distance of L0.end L1.end
  measures "d4" distance of L0.start L3
  measures "d5" distance of L4.end L5.end
  measures "d6" distance of L0.end L6
  measures "d8" diameter of A0
  measures "d9" distance of L0.start A0.centre
revolve "Revolve1" add sketch "Sketch1" angle 360 about axis through (0, 0, 1.75) along (0, 0, 1) contours L0 L1 L2 L3 L4 L5 L6 L7
extrude "Extrude1" cut sketch "Sketch1" against normal blind 17 contours A0
equation "d1 = ( 5 / 2 ) * 1 mm"
equation "d2 = ( 16 / 2 ) * 1 mm"
equation "d4 = ( 20 * 2 / PI ) * 1 mm / 2"

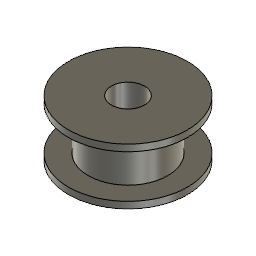
design "y axis pulley idler"
Autodesk Fusion 360 part; units mm, degrees
sketch "Sketch1" plane through (0, 0, 0) normal (0, 0, 1) x (1, 0, 0)
  circle A0 centre (0, 0) radius 9
  dimension "d1" = 18
  constraint coincident A0.centre origin
  measures "d1" diameter of A0
extrude "Extrude1" add sketch "Sketch1" along normal blind 1
sketch "Sketch2" plane through (0, 0, 1) normal (0, 0, 1) x (-1, 0, 0)
  circle A0 centre (0, 0) radius 9
  circle A1 centre (0, 0) radius 6
  dimension "d4" = 12
  constraint coincident A0.centre A1.centre
  measures "d4" diameter of A1
extrude "Extrude2" add sketch "Sketch2" along normal blind 6.5 contours A1
sketch "Sketch3" plane through (0, 0, 7.5) normal (0, 0, 1) x (-1, 0, 0)
  circle A0 centre (0, 0) radius 6
  circle A1 centre (0, 0) radius 9
  dimension "d7" = 18
  constraint coincident A0.centre A1.centre
  measures "d7" diameter of A1
extrude "Extrude3" add sketch "Sketch3" along normal blind 1 contours A0 | A1
sketch "Sketch4" plane through (0, 0, 8.5) normal (0, 0, 1) x (-1, 0, 0)
  circle A0 centre (0, 0) radius 9
  circle A1 centre (0, 0) radius 2.5
  dimension "d10" = 5
  constraint coincident A0.centre A1.centre
  measures "d10" diameter of A1
extrude "Extrude4" cut sketch "Sketch4" against normal up to surface (8.5 mm away) contours A1
